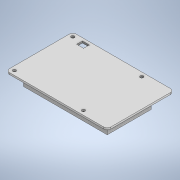
# Autodesk Inventor part: Pi4BatteryBoard_Mockup
Saved by Autodesk Inventor 2021 (Build 250183000, 183)
## iProperties
Created: 2021-04-19
Part Number: Pi4BatteryBoard_Mockup
Material: Generic
Document SubType Name: Modeling
Designer: trent
Density: 1 g/cm^3
Appearance: Default
Author: trent
Autodesk Inventor part; units mm, degrees
ref_plane "YZ Plane" through (0, 0, 0) normal (1, 0, 0) x (0, 1, 0)
ref_plane "XZ Plane" through (0, 0, 0) normal (0, 1, 0) x (-1, 0, 0)
ref_plane "XY Plane" through (0, 0, 0) normal (0, 0, 1) x (1, 0, 0)
sketch "Sketch1" plane through (0, 0, 0) normal (0, 1, 0) x (-1, 0, 0)
  line L0 (-3, 0) -> (-82, 0)
  line L1 (-85, -3) -> (-85, -53)
  line L2 (-82, -56) -> (-3, -56)
  line L3 (0, -53) -> (0, -3)
  arc A0 (-3, -56) -> (0, -53) centre (-3, -53) ccw
  arc A1 (0, -3) -> (-3, 0) centre (-3, -3) ccw
  arc A2 (-82, 0) -> (-85, -3) centre (-82, -3) ccw
  arc A3 (-85, -53) -> (-82, -56) centre (-82, -53) ccw
  circle A4 centre (-3.5, -52.5) radius 1.35
  circle A5 centre (-3.5, -3.5) radius 1.35
  circle A6 centre (-61.5, -52.5) radius 1.35
  circle A7 centre (-61.5, -3.5) radius 1.35
  point P0 (0, 0)
  point P1 (-85, -56)
  point P2 (-85, 0)
  point P3 (0, -56)
  dimension "d0" = 85
  dimension "d1" = 56
  dimension "d2" = 3
  dimension "d9" = 2.7
  dimension "d10" = 2.7
  dimension "d15" = 2.7
  dimension "d16" = 2.7
  dimension "d140" = 58
  dimension "d141" = 58
  dimension "d142" = 49
  dimension "d143" = 3.5
  constraints: 8 centre point, 8 end point, 8 point on circle, 8 point on line, 8 tangent, 3 equal radius, 2 parallel, 1 horizontal, 1 perpendicular
  measures "d0" distance of point (-85, -56) point (0, -56)
  measures "d1" distance of point (-85, 0) point (-85, -56)
  measures "d2" radius of A0
  measures "d9" diameter of A4
  measures "d10" diameter of A5
  measures "d15" diameter of A6
  measures "d16" diameter of A7
  measures "d140" distance of A6.centre A4.centre
  measures "d141" distance of A5.centre A7.centre
  measures "d142" distance of A4.centre A5.centre
  measures "d143" distance from line of L0 A5.centre
extrude "Extrusion1" add sketch "Sketch1" along normal blind 1.5
sketch "Sketch12" plane through (0, 0, 0) normal (0, -1, 0) x (1, 0, 0)
  line L0 (5, -9.5) -> (75.5, -9.5)
  line L1 (75.5, -9.5) -> (75.5, -46.5)
  line L2 (75.5, -46.5) -> (5, -46.5)
  line L3 (5, -46.5) -> (5, -9.5)
  line L4 (82, -56) -> (3, -56) projected
  line L5 (85, -3) -> (85, -53) projected
  line L6 (3, 0) -> (82, 0) projected
  line L7 (0, -53) -> (0, -3) projected
  point P0 (0, 0)
  dimension "d152" = 9.5
  dimension "d153" = 9.5
  dimension "d154" = 9.5
  dimension "d155" = 5
  constraints: 8 end point, 2 parallel, 1 horizontal, 1 perpendicular
  measures "d152" distance between parallel lines of L4 L2
  measures "d153" distance between parallel lines of L5 L1
  measures "d154" distance between parallel lines of L6 L0
  measures "d155" distance between parallel lines of L7 L3
extrude "Extrusion12" add sketch "Sketch12" along normal blind 12.25
sketch "Sketch13" plane through (0, 0, 0) normal (0, -1, 0) x (1, 0, 0)
  line L0 (10.5, -53.65) -> (16.35, -53.65)
  line L1 (16.35, -53.65) -> (16.35, -48.8)
  line L2 (16.35, -48.8) -> (10.5, -48.8)
  line L3 (10.5, -48.8) -> (10.5, -53.65)
  line L4 (0, -53) -> (0, -3) projected
  line L5 (82, -56) -> (3, -56) projected
  point P0 (0, 0)
  dimension "d146" = 10.5
  dimension "d147" = 2.35
  dimension "d148" = 4.85
  dimension "d149" = 5.85
  constraints: 8 end point, 2 parallel, 1 horizontal, 1 perpendicular
  measures "d146" distance between parallel lines of L4 L3
  measures "d147" distance between parallel lines of L5 L0
  measures "d148" distance of L2.end L0.start
  measures "d149" distance of L0.start L0.end
extrude "Extrusion13" cut sketch "Sketch13" against normal up to next
body "Solid1"
